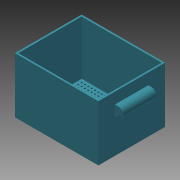
# Autodesk Inventor part: 集肉皿
Saved by Autodesk Inventor 2015 (Build 190159000, 159)
## iProperties
Created: 2017-05-22
Part Number: 集肉皿
Material: 常规
Document SubType Name: Modeling
Designer: Administrator
Density: 1 g/cm^3
Appearance: 灰蓝色
Author: Administrator
Autodesk Inventor part; units mm, degrees
ref_plane "YZ Plane" through (0, 0, 0) normal (1, 0, 0) x (0, 1, 0)
ref_plane "XZ Plane" through (0, 0, 0) normal (0, 1, 0) x (-1, 0, 0)
ref_plane "XY Plane" through (0, 0, 0) normal (0, 0, 1) x (1, 0, 0)
sketch "草图1" plane through (0, 0, 0) normal (0, 0, 1) x (1, 0, 0)
  line L0 (0, 0) -> (150, 0)
  line L1 (150, 0) -> (150, -120)
  line L2 (150, -120) -> (0, -120)
  line L3 (0, -120) -> (0, 0)
  dimension "d0" = 150
  dimension "d1" = 120
  constraints: 8 end point, 2 parallel, 1 horizontal, 1 perpendicular
  measures "d0" distance of L1.end L2.end
  measures "d1" distance of L2.end L0.start
extrude "拉伸1" add sketch "草图1" along normal blind 100
shell "抽壳1" thickness 3 removed faces 1 at (50, -40, 100)
sketch "草图2" plane through (3, -3, 3) normal (0, 0, 1) x (1, 0, 0)
  circle A0 centre (6, -6) radius 1.5
  line L0 (0, 0) -> (144, 0) projected
  line L1 (0, -114) -> (0, 0) projected
  point P0 (-3, 3)
  dimension "d5" = 3
  dimension "d6" = 6
  dimension "d7" = 6
  constraints: 1 centre point
  measures "d5" diameter of A0
  measures "d6" distance from line of A0.centre L0
  measures "d7" distance from line of L1 A0.centre
extrude "拉伸2" cut sketch "草图2" against normal through all
pattern_linear "矩形阵列1" count 18 spacing 6 along (0, -1, 0) of "拉伸2"
pattern_linear "矩形阵列2" count 23 spacing 6 along (1, 0, 0) of "拉伸2", "矩形阵列1"
sketch "草图3" plane through (150, -120, 0) normal (1, 0, 0) x (0, 0, -1)
  line L0 (-80, 30) -> (-60, 30)
  line L1 (-60, 30) -> (-60, 90)
  line L2 (-60, 90) -> (-80, 90)
  line L3 (-80, 90) -> (-80, 30)
  line L4 (0, 120) -> (-100, 120) projected
  line L5 (-100, 0) -> (-100, 120) projected
  dimension "d16" = 60
  dimension "d17" = 20
  dimension "d18" = 30
  dimension "d19" = 20
  constraints: 8 end point, 2 parallel, 1 horizontal, 1 perpendicular
  measures "d16" distance of L2.end L0.start
  measures "d17" distance of L1.end L2.end
  measures "d18" distance between parallel lines of L4 L2
  measures "d19" distance between parallel lines of L5 L3
extrude "拉伸3" add sketch "草图3" along normal blind 15
sketch "草图4" plane through (150, -90, 60) normal (0, -1, 0) x (1, 0, 0)
  circle A0 centre (7.5, 0) radius 7.5
  line L0 (0, 0) -> (15, 0) projected
  point P0 (-150, -60)
  dimension "d22" = 15
  constraints: 1 centre point, 1 coincident, 1 midpoint
  measures "d22" diameter of A0
extrude "拉伸4" cut sketch "草图4" against normal blind 60
pattern_linear "矩形阵列3" count 2 spacing 165 along (-1, 0, 0) of "拉伸4", "拉伸3"
fillet "圆角1" radius 2 2 edges at (165, -60, 60) (-15, -60, 60)
fillet "圆角2" radius 10 2 edges at (-15, -60, 80) (165, -60, 80)
